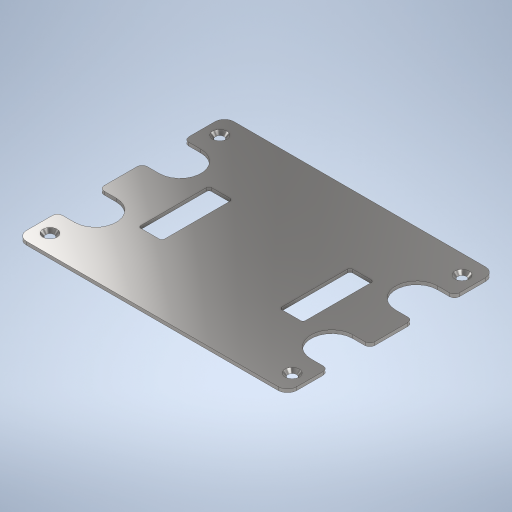
# Autodesk Inventor part: spacer
Saved by Autodesk Inventor 2023 (Build 270158000, 158)
## iProperties
Created: 2021-07-16
Part Number: spacer
Material: Stainless Steel
Document SubType Name: Modeling
Designer: Caleb
Density: 8 g/cm^3
Appearance: Semi-Polished
Author: Caleb
Autodesk Inventor part; units mm, degrees
ref_plane "YZ Plane" through (0, 0, 0) normal (1, 0, 0) x (0, 1, 0)
ref_plane "XZ Plane" through (0, 0, 0) normal (0, 1, 0) x (-1, 0, 0)
ref_plane "XY Plane" through (0, 0, 0) normal (0, 0, 1) x (1, 0, 0)
sketch "Sketch1" plane through (0, 0, 0) normal (0, 1, 0) x (-1, 0, 0)
  line L0 (-26.75, 22.05) -> (26.75, 22.05)
  line L1 (28.75, 20.05) -> (28.75, -20.05)
  line L2 (26.75, -22.05) -> (-26.75, -22.05)
  line L3 (-28.75, -20.05) -> (-28.75, 20.05)
  line L4 (-28.75, 22.05) -> (28.75, -22.05) construction
  line L5 (28.75, 22.05) -> (-28.75, -22.05) construction
  arc A0 (28.75, 20.05) -> (26.75, 22.05) centre (26.75, 20.05) ccw
  arc A1 (26.75, -22.05) -> (28.75, -20.05) centre (26.75, -20.05) ccw
  arc A2 (-28.75, -20.05) -> (-26.75, -22.05) centre (-26.75, -20.05) ccw
  arc A3 (-26.75, 22.05) -> (-28.75, 20.05) centre (-26.75, 20.05) ccw
  point P0 (0, 0)
  dimension "d0" = 44.1
  dimension "d1" = 57.5
  dimension "d2" = 2
  constraints: 12 end point, 8 point on circle, 8 point on line, 8 tangent, 4 centre point, 3 equal radius, 2 midpoint, 2 parallel, 1 horizontal, 1 perpendicular
  measures "d0" distance of L5.start L4.end
  measures "d1" distance of L4.end L5.end
  measures "d2" radius of A0
extrude "Extrusion1" add sketch "Sketch1" along normal blind 0.7
sketch "Sketch2" plane through (0, 0.7, 0) normal (0, 1, 0) x (1, 0, 0)
  point P0 (0, 0)
  point P1 (-25.75, 18.05)
  point P2 (25.75, 18.05)
  point P3 (-25.75, -18.05)
  point P4 (25.75, -18.05)
  dimension "d76" = 51.5
  dimension "d77" = 36.1
  dimension "d78" = 18.05
  dimension "d79" = 25.75
  constraints: 2 horizontal alignment, 2 vertical alignment
  measures "d76" distance of point (25.75, 18.05) point (-25.75, 18.05)
  measures "d77" distance of point (-25.75, -18.05) point (-25.75, 18.05)
  measures "d78" vertical distance of point (-25.75, 18.05) point (0, 0)
  measures "d79" horizontal distance of point (-25.75, 18.05) point (0, 0)
hole "Hole1" at (-25.75, 0.7, -18.05) at (25.75, 0.7, -18.05) at (-25.75, 0.7, 18.05) at (25.75, 0.7, 18.05) direction (0, -1, 0) diameter 1.778 end through all countersink diameter 3.023 countersink angle 82 clearance for "Flat Head Machine Screw (82)" size "#0" standard "Ansi Unified Screw Threads"
sketch "Sketch3" plane through (0, 0.7, 0) normal (0, 1, 0) x (1, 0, 0)
  line L0 (-13, -7.5) -> (-17, -7.5)
  line L1 (-17.5, -7) -> (-17.5, 7)
  line L2 (-17, 7.5) -> (-13, 7.5)
  line L3 (-12.5, -7.5) -> (-17.5, 7.5) construction
  line L4 (-17.5, -7.5) -> (-12.5, 7.5) construction
  line L5 (17, -7.5) -> (13, -7.5)
  line L6 (13, 7.5) -> (17, 7.5)
  line L7 (17.5, 7) -> (17.5, -7)
  line L8 (17.5, -7.5) -> (12.5, 7.5) construction
  line L9 (12.5, -7.5) -> (17.5, 7.5) construction
  arc A0 (-17.5, -7) -> (-17, -7.5) centre (-17, -7) ccw
  arc A1 (-17, 7.5) -> (-17.5, 7) centre (-17, 7) ccw
  arc A2 (17, -7.5) -> (17.5, -7) centre (17, -7) ccw
  arc A3 (17.5, 7) -> (17, 7.5) centre (17, 7) ccw
  line L10 (-12.5, 7) -> (-12.5, -7)
  arc A4 (-13, -7.5) -> (-12.5, -7) centre (-13, -7) ccw
  arc A5 (-12.5, 7) -> (-13, 7.5) centre (-13, 7) ccw
  line L11 (12.5, 7) -> (12.5, -7)
  arc A6 (12.5, -7) -> (13, -7.5) centre (13, -7) ccw
  arc A7 (13, 7.5) -> (12.5, 7) centre (13, 7) ccw
  point P0 (0, 0)
  point P1 (-15, 0)
  point P2 (15, 0)
  point P3 (-15, 0)
  point P4 (15, 0)
  point P5 (-15, 0)
  dimension "d18" = 15
  dimension "d21" = 5
  dimension "d72" = 30
  dimension "d73" = 15
  dimension "d85" = 0.5
  dimension "d88" = 0.5
  dimension "d89" = 0.5
  dimension "d90" = 0.5
  dimension "d91" = 5
  dimension "d92" = 15
  constraints: 24 end point, 20 point on line, 16 point on circle, 16 tangent, 8 centre point, 7 midpoint, 3 parallel, 2 equal radius, 2 horizontal, 2 horizontal alignment, 2 vertical, 1 coincident, 1 collinear, 1 perpendicular
  measures "d18" distance of L4.start L3.end
  measures "d21" distance of L3.start L4.start
  measures "d72" distance of point (15, 0) point (-15, 0)
  measures "d73" distance of point (-15, 0) point (0, 0)
  measures "d85" radius of A0
  measures "d88" radius of A1
  measures "d89" radius of A4
  measures "d90" radius of A6
  measures "d91" distance between parallel lines of L7 L11
  measures "d92" distance between parallel lines of L6 L5
extrude "Extrusion2" cut sketch "Sketch3" against normal through all
sketch "Sketch8" plane through (0, 0.7, 0) normal (0, 1, 0) x (1, 0, 0)
  circle A0 centre (25.15, -9) radius 4.445
  circle A1 centre (25.15, 9) radius 4.445
  line L0 (28.75, -20.05) -> (28.75, 20.05) projected
  line L1 (0, -25.8162) -> (0, 35.4603)
  line L2 (25.15, -13.445) -> (28.75, -13.445)
  line L3 (28.75, -13.445) -> (28.75, -11.6073)
  line L4 (28.75, -20.05) -> (28.75, 20.05) projected
  line L5 (25.15, -4.555) -> (28.75, -4.555)
  line L6 (28.75, -4.555) -> (28.75, -6.3927)
  line L7 (25.15, 4.555) -> (28.75, 4.555)
  line L8 (25.15, 13.445) -> (28.75, 13.445)
  line L9 (28.75, 4.555) -> (28.75, 6.3927)
  line L10 (28.75, 13.445) -> (28.75, 11.6073)
  circle A2 centre (-25.15, -9) radius 4.445
  circle A3 centre (-25.15, 9) radius 4.445
  line L11 (-28.75, -20.05) -> (-28.75, 20.05)
  line L12 (-25.15, -13.445) -> (-28.75, -13.445)
  line L13 (-28.75, -13.445) -> (-28.75, -11.6073)
  line L14 (-28.75, -20.05) -> (-28.75, 20.05)
  line L15 (-25.15, -4.555) -> (-28.75, -4.555)
  line L16 (-28.75, -4.555) -> (-28.75, -6.3927)
  line L17 (-25.15, 4.555) -> (-28.75, 4.555)
  line L18 (-25.15, 13.445) -> (-28.75, 13.445)
  line L19 (-28.75, 4.555) -> (-28.75, 6.3927)
  line L20 (-28.75, 13.445) -> (-28.75, 11.6073)
  point P0 (0, 0)
  point P1 (28.75, -11.6073)
  point P2 (-28.75, 11.6073)
  point P3 (28.75, 11.6073)
  dimension "d93" = 8.89
  dimension "d94" = 9
  dimension "d95" = 8.89
  dimension "d96" = 9
  dimension "d97" = 3.6
  constraints: 36 end point, 16 point on circle, 16 symmetric about line, 5 point on line, 4 centre point, 3 perpendicular, 3 tangent, 2 vertical, 1 horizontal, 1 vertical alignment, 16 other
  measures "d93" diameter of A0
  measures "d94" vertical distance of A0.centre point (0, 0)
  measures "d95" diameter of A1
  measures "d96" vertical distance of point (0, 0) A1.centre
  measures "d97" distance from line of L0 A0.centre
extrude "Extrusion5" cut sketch "Sketch8" against normal through all contours A0 L0 | L0 A0 | A0 L5 L0 | L0 L2 A0 | A1 L0 | L0 A1 | A1 L8 L0 | L0 L7 A1 | A2 L11 | A2 L11 L15 | L12 L11 A2 | A3 L11 | A3 L11 L18 | L17 L11 A3 picked at (-26.0683, -9) picked at (-26.0683, 9)
fillet "Fillet2" radius 1 8 edges at (28.75, 0.35, 13.445) (28.75, 0.35, 4.555) (28.75, 0.35, -4.555) (28.75, 0.35, -13.445) (-28.75, 0.35, -13.445) (-28.75, 0.35, -4.555) (-28.75, 0.35, 4.555) (-28.75, 0.35, 13.445)
equation "\"d73\" = 0.5 * d72"
equation "\"d88\" = d85"
equation "\"d89\" = d85"
equation "\"d90\" = d85"
equation "\"d91\" = d21"
equation "\"d92\" = d18"
equation "\"d95\" = d93"
equation "\"d96\" = d94"
body "Solid1"
